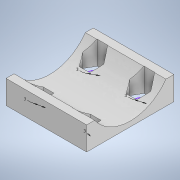
# Autodesk Inventor part: держатель_гаек
Saved by Autodesk Inventor 2020 (Build 240168000, 168)
## iProperties
Created: 2022-07-30
Part Number: держатель_гаек
Material: Типовые
Document SubType Name: Modeling
Designer: akapu
Density: 1 g/cm^3
Appearance: По умолчанию
Author: akapu
Autodesk Inventor part; units mm, degrees
ref_plane "YZ Plane" through (0, 0, 0) normal (1, 0, 0) x (0, 1, 0)
ref_plane "XZ Plane" through (0, 0, 0) normal (0, 1, 0) x (-1, 0, 0)
ref_plane "XY Plane" through (0, 0, 0) normal (0, 0, 1) x (1, 0, 0)
sketch "Эскиз1" plane through (0, 0, 0) normal (0, 1, 0) x (-1, 0, 0)
  line L0 (7, -8) -> (-7, -8)
  line L1 (-7, -8) -> (-7, 8)
  line L2 (-7, 8) -> (7, 8)
  line L3 (7, 8) -> (7, -8)
  circle A0 centre (7, 8) radius 1.6
  circle A1 centre (7, -8) radius 1.6
  circle A2 centre (-7, -8) radius 1.6
  circle A3 centre (-7, 8) radius 1.6
  line L4 (7, 8) -> (7, 5.3)
  line L5 (7, -8) -> (7, -5.3)
  line L6 (-7, -8) -> (-7, -5.3)
  line L7 (-7, 8) -> (-7, 5.3)
  line L8 (5.4412, 5.3) -> (3.8823, 8)
  line L9 (3.8823, 8) -> (5.4412, 10.7)
  line L10 (5.4412, 10.7) -> (8.5588, 10.7)
  line L11 (8.5588, 10.7) -> (10.1177, 8)
  line L12 (10.1177, 8) -> (8.5588, 5.3)
  line L13 (8.5588, 5.3) -> (5.4412, 5.3)
  line L14 (8.5588, -5.3) -> (10.1177, -8)
  line L15 (10.1177, -8) -> (8.5588, -10.7)
  line L16 (8.5588, -10.7) -> (5.4412, -10.7)
  line L17 (5.4412, -10.7) -> (3.8823, -8)
  line L18 (3.8823, -8) -> (5.4412, -5.3)
  line L19 (5.4412, -5.3) -> (8.5588, -5.3)
  line L20 (-5.4412, -5.3) -> (-3.8823, -8)
  line L21 (-3.8823, -8) -> (-5.4412, -10.7)
  line L22 (-5.4412, -10.7) -> (-8.5588, -10.7)
  line L23 (-8.5588, -10.7) -> (-10.1177, -8)
  line L24 (-10.1177, -8) -> (-8.5588, -5.3)
  line L25 (-8.5588, -5.3) -> (-5.4412, -5.3)
  line L26 (-8.5588, 5.3) -> (-10.1177, 8)
  line L27 (-10.1177, 8) -> (-8.5588, 10.7)
  line L28 (-8.5588, 10.7) -> (-5.4412, 10.7)
  line L29 (-5.4412, 10.7) -> (-3.8823, 8)
  line L30 (-3.8823, 8) -> (-5.4412, 5.3)
  line L31 (-5.4412, 5.3) -> (-8.5588, 5.3)
  line L32 (-12, 8) -> (-12, 13)
  line L33 (-12, 13) -> (-7, 13)
  line L34 (-12, 13) -> (12, 13)
  line L35 (12, 13) -> (12, -13)
  line L36 (12, -13) -> (-12, -13)
  line L37 (-12, -13) -> (-12, 13)
  point P0 (0, 0)
  dimension "d2" = 14
  dimension "d3" = 16
  dimension "d4" = 3.2
  dimension "d5" = 3.2
  dimension "d6" = 3.2
  dimension "d7" = 3.2
  dimension "d8" = 2.7
  dimension "d9" = 2.7
  dimension "d10" = 2.7
  dimension "d11" = 2.7
  dimension "d12" = 5
  dimension "d13" = 5
  dimension "d14" = 24
  dimension "d15" = 26
  constraints: 76 end point, 7 coincident, 4 centre point, 4 midpoint, 4 parallel, 4 point on line, 2 horizontal, 2 perpendicular, 39 other
  measures "d2" distance of L1.end L2.end
  measures "d3" distance of L0.end L1.end
  measures "d4" diameter of A0
  measures "d5" diameter of A1
  measures "d6" diameter of A2
  measures "d7" diameter of A3
  measures "d8" distance of L4.start L4.end
  measures "d9" distance of L5.start L5.end
  measures "d10" distance of L6.start L6.end
  measures "d11" distance of L7.start L7.end
  measures "d12" distance of L32.end L33.end
  measures "d13" distance of L32.start L32.end
  measures "d14" distance of L35.end L36.end
  measures "d15" distance of L34.end L35.end
extrude "Выдавливание1" add sketch "Эскиз1" along normal blind 20 contours L0 L20 L25 L1 L31 L30 L2 L8 L13 L3 L19 L18 | L32 L33 L34 L35 L36 L37
sketch "Эскиз2" plane through (12, 0, 13) normal (1, 0, 0) x (0, 0, -1)
  line L0 (13, 0) -> (13, 14.5)
  circle A0 centre (13, 14.5) radius 12.5
  line L1 (0, 0) -> (0, 20) projected
  line L2 (0, 0) -> (0, 7)
  line L3 (26, 0) -> (26, 20) projected
  line L4 (26, 20) -> (0, 20) projected
  line L5 (0, 7) -> (26, 7)
  line L6 (26, 7) -> (26, 20)
  line L7 (26, 20) -> (0, 20)
  line L8 (0, 20) -> (0, 7)
  circle A1 centre (13, 14.5) radius 13
  point P0 (23, 7)
  point P1 (24.225, 20)
  point P2 (3, 7)
  point P3 (1.775, 20)
  point P4 (24.7792, 20)
  point P5 (1.2208, 20)
  point P6 (2.3816, 7)
  point P7 (23.6184, 7)
  dimension "d18" = 14.5
  dimension "d19" = 25
  dimension "d22" = 7
  dimension "d23" = 26
  constraints: 12 end point, 2 centre point, 2 coincident, 2 parallel, 1 horizontal, 1 perpendicular, 1 point on line, 1 vertical
  measures "d18" distance of L0.start L0.end
  measures "d19" diameter of A0
  measures "d22" distance of L1.start L2.end
  measures "d23" diameter of A1
extrude "Выдавливание2" cut sketch "Эскиз2" against normal blind 24
sketch "Эскиз3" plane through (0, 0, 0) normal (0, -1, 0) x (1, 0, 0)
  circle A0 centre (7, 8) radius 1.5
  circle A1 centre (7, -8) radius 1.5
  circle A2 centre (-7, -8) radius 1.5
  circle A3 centre (-7, 8) radius 1.5
  point P0 (0, 0)
  dimension "d24" = 3
  dimension "d25" = 3
  dimension "d26" = 3
  dimension "d27" = 3
  constraints: 4 centre point
  measures "d24" diameter of A0
  measures "d25" diameter of A1
  measures "d26" diameter of A2
  measures "d27" diameter of A3
